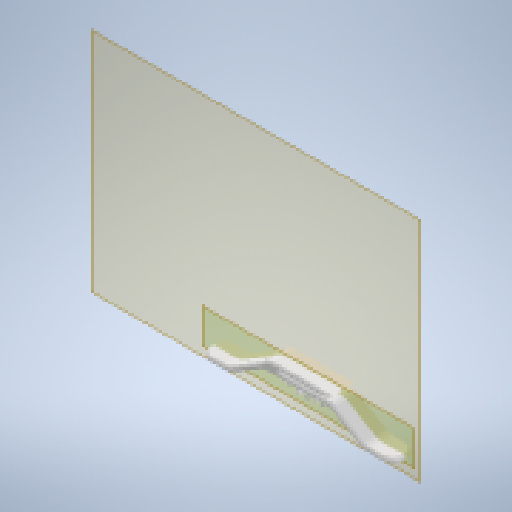
# Autodesk Inventor part: cable-hanger
Saved by Autodesk Inventor 2023 (Build 270158030, 158C)
## iProperties
Created: 2024-09-24
Part Number: cable-hanger
Material: Generic
Document SubType Name: Modeling
Designer: Imogen Heard
Density: 1 g/cm^3
Appearance: Default
Author: Imogen Heard
Autodesk Inventor part; units mm, degrees
ref_plane "YZ Plane" through (0, 0, 0) normal (1, 0, 0) x (0, 1, 0)
ref_plane "XZ Plane" through (0, 0, 0) normal (0, 1, 0) x (-1, 0, 0)
ref_plane "XY Plane" through (0, 0, 0) normal (0, 0, 1) x (1, 0, 0)
sketch "Sketch1" plane through (0, 0, 0) normal (0, 0, 1) x (1, 0, 0)
  line L0 (-0.831, -6.5) -> (-20.831, -6.5)
  line L1 (-20.831, -6.5) -> (-20.831, -3.5)
  line L2 (-20.831, -3.5) -> (0, -3.5)
  line L3 (0, -3.5) -> (20, -15.5)
  line L4 (20, -15.5) -> (36.169, -15.5)
  line L5 (36.169, -15.5) -> (36.169, -18.5)
  line L6 (36.169, -18.5) -> (19.169, -18.5)
  line L7 (19.169, -18.5) -> (-0.831, -6.5)
  line L8 (-40.831, -6.5) -> (-20.831, -6.5)
  line L9 (-20.831, -3.5) -> (-41.6619, -3.5)
  line L10 (-41.6619, -3.5) -> (-61.6619, -15.5)
  line L11 (-61.6619, -15.5) -> (-77.831, -15.5)
  line L12 (-77.831, -15.5) -> (-77.831, -18.5)
  line L13 (-77.831, -18.5) -> (-60.831, -18.5)
  line L14 (-60.831, -18.5) -> (-40.831, -6.5)
  line L15 (-41.6619, -3.5) -> (-31.6619, -3.5)
  line L16 (-31.6619, -3.5) -> (-31.6619, -2)
  line L17 (-31.6619, -2) -> (-41.6619, -2)
  line L18 (-41.6619, -2) -> (-41.6619, -3.5)
  line L19 (-41.6619, -2) -> (0, -2)
  line L20 (0, -2) -> (0, 0)
  line L21 (0, 0) -> (-41.6619, 0)
  line L22 (-41.6619, 0) -> (-41.6619, -2)
  point P0 (65.831, 133)
  point P1 (105.831, 133)
  point P2 (106.6619, 130)
  point P3 (96.6619, 130)
  point P4 (96.6619, 128.5)
  dimension "d0" = 3
  dimension "d1" = 3
  dimension "d2" = 3
  dimension "d3" = 17
  dimension "d4" = -20
  dimension "d5" = -12
  dimension "d6" = 20
  dimension "d7" = 114
  dimension "d8" = 20
  dimension "d9" = -20
  dimension "d10" = 17
  dimension "d11" = 2
  dimension "d12" = 1.5
  dimension "d13" = 10
  constraints: 46 end point, 7 symmetric about line, 6 parallel, 5 perpendicular, 2 coincident, 1 horizontal alignment, 1 vertical alignment
  measures "d0" distance between parallel lines of L2 L0
  measures "d1" distance between parallel lines of L3 L7
  measures "d2" distance between parallel lines of L4 L6
  measures "d3" distance from line of L5 L6.end
  measures "d4" horizontal distance of L0.start L6.end
  measures "d5" vertical distance of L0.start L6.end
  measures "d6" distance of L0.start L0.end
  measures "d7" distance between parallel lines of L12 L5
  measures "d8" distance from line of L8.start L1
  measures "d9" horizontal distance of L13.end L14.end
  measures "d10" distance of L12.end L13.end
  measures "d11" distance between parallel lines of L21 L19
  measures "d12" distance between parallel lines of L19 L9
  measures "d13" distance between parallel lines of L16 L22
extrude "Extrusion1" add sketch "Sketch1" along normal blind 15
fillet "Fillet1" radius 7.5 4 edges at (-77.831, -17, 0) (-77.831, -17, 15) (36.169, -17, 15) (36.169, -17, 0)
fillet "Fillet2" radius 10 9 edges at (-41.6619, 0, 7.5) (-61.6619, -15.5, 7.5) (-60.831, -18.5, 7.5) (-40.831, -6.5, 7.5) (-0.831, -6.5, 7.5) (19.169, -18.5, 7.5) (20, -15.5, 7.5) (0, -3.5, 7.5) (0, -2, 7.5)
chamfer "Chamfer1" distance 1 angle 45 50 edges at (-20.831, -6.5, 0) (-0.9315, -6.8629, 0) (9.169, -12.5, 0) (19.2696, -18.1371, 0) (25.304, -18.5, 0) (33.9724, -18.5, 2.1967) (36.169, -18.5, 7.5) (33.9724, -18.5, 12.8033) (25.304, -18.5, 15) (19.2696, -18.1371, 15) (9.169, -12.5, 15) (-0.9315, -6.8629, 15) (-20.831, -6.5, 15) (-40.7304, -6.8629, 15) (-50.831, -12.5, 15) (-60.9315, -18.1371, 15) (-66.9659, -18.5, 15) (-75.6343, -18.5, 2.1967) (-77.831, -18.5, 7.5) (-75.6343, -18.5, 12.8033) (-66.9659, -18.5, 0) (-60.9315, -18.1371, 0) (-50.831, -12.5, 0) (-40.7304, -6.8629, 0) (-50.4743, -8.7875, 15) (-61.7624, -15.1371, 15) (-67.3814, -15.5, 15) (-75.6343, -15.5, 2.1967) (-77.831, -15.5, 7.5) (-75.6343, -15.5, 12.8033) (-67.3814, -15.5, 0) (-61.7624, -15.1371, 0) (-50.4743, -8.7875, 0) (-38.2459, -0.917, 15) (-17.0313, 0, 15) (-38.2459, -0.917, 0) (-17.0313, 0, 0) (25.7195, -15.5, 15) (20.1005, -15.1371, 15) (10, -9.5, 15) (-0.1005, -3.8629, 15) (-17.2159, -3.5, 15) (33.9724, -15.5, 2.1967) (36.169, -15.5, 7.5) (33.9724, -15.5, 12.8033) (25.7195, -15.5, 0) (20.1005, -15.1371, 0) (10, -9.5, 0) (-0.1005, -3.8629, 0) (-17.2159, -3.5, 0)
ref_plane "Work Plane1" through (0, 0, 7.5) normal (0, 0, 1) x (1, 0, 0)
sketch "Sketch2" plane through (0, 0, 7.5) normal (0, 0, 1) x (1, 0, 0)
  circle A0 centre (-135.4999, 85.8508) radius 2.5
  circle A1 centre (-134.65, 75.8508) radius 1.65
  line L0 (-133, 103.0611) -> (-133, 68.6008)
  circle A2 centre (-135, 95.8508) radius 2
  circle A3 centre (-134.65, 75.8508) radius 2.85
  circle A4 centre (-135.4999, 85.8508) radius 3.7
  circle A5 centre (-135, 95.8508) radius 3.2
  line L1 (-137.9999, 75.0258) -> (-135.6676, 75.0258)
  line L2 (-135.6676, 75.0258) -> (-135.6676, 76.6758)
  line L3 (-135.6676, 76.6758) -> (-137.9999, 76.6758)
  line L4 (-137.9999, 76.6758) -> (-137.9999, 75.0258)
  line L5 (-139.843, 84.6008) -> (-137.5, 84.6008)
  line L6 (-137.5, 84.6008) -> (-137.5, 87.1008)
  line L7 (-137.5, 87.1008) -> (-139.843, 87.1008)
  line L8 (-139.843, 87.1008) -> (-139.843, 84.6008)
  line L9 (-138.6715, 94.8508) -> (-136.0812, 94.8508)
  line L10 (-136.0812, 94.8508) -> (-136.0812, 96.8508)
  line L11 (-136.0812, 96.8508) -> (-138.6715, 96.8508)
  line L12 (-138.6715, 96.8508) -> (-138.6715, 94.8508)
  circle A6 centre (-135.4999, 85.8508) radius 2.5
  circle A7 centre (-134.65, 75.8508) radius 1.65
  line L13 (-133, 103.0611) -> (-133, 68.6008)
  circle A8 centre (-135, 95.8508) radius 2
  circle A9 centre (-134.65, 75.8508) radius 2.85
  circle A10 centre (-135.4999, 85.8508) radius 3.7
  circle A11 centre (-135, 95.8508) radius 3.2
  line L14 (-137.9999, 75.0258) -> (-135.6676, 75.0258)
  line L15 (-135.6676, 75.0258) -> (-135.6676, 76.6758)
  line L16 (-135.6676, 76.6758) -> (-137.9999, 76.6758)
  line L17 (-137.9999, 76.6758) -> (-137.9999, 75.0258)
  line L18 (-139.843, 84.6008) -> (-137.5, 84.6008)
  line L19 (-137.5, 84.6008) -> (-137.5, 87.1008)
  line L20 (-137.5, 87.1008) -> (-139.843, 87.1008)
  line L21 (-139.843, 87.1008) -> (-139.843, 84.6008)
  line L22 (-138.6715, 94.8508) -> (-136.0812, 94.8508)
  line L23 (-136.0812, 94.8508) -> (-136.0812, 96.8508)
  line L24 (-136.0812, 96.8508) -> (-138.6715, 96.8508)
  line L25 (-138.6715, 96.8508) -> (-138.6715, 94.8508)
  circle A12 centre (-11.331, -9) radius 2.5
  circle A13 centre (-20.831, -9.5) radius 3
  circle A14 centre (-30.331, -8.5) radius 2
  line L26 (28.669, -16.5) -> (28.669, -16.5) projected
  line L27 (28.669, -16.5) -> (28.669, -17.5) projected
  line L28 (28.669, -17.5) -> (28.669, -17.5) projected
  line L29 (28.669, -17.5) -> (28.669, -16.5) projected
  line L30 (22.7698, -16.5) -> (28.669, -16.5) projected
  arc A15 (17.1104, -14.9324) -> (22.7698, -16.5) centre (22.7698, -5.5) ccw projected
  line L31 (1.8606, -5.7826) -> (17.1104, -14.9324) projected
  arc A16 (1.8606, -5.7826) -> (-2.7698, -4.5) centre (-2.7698, -13.5) ccw projected
  line L32 (-31.6619, -4.5) -> (-2.7698, -4.5) projected
  line L33 (-31.6619, -4.5) -> (-31.6619, -2) projected
  line L34 (-31.6619, -2) -> (-6, -2) projected
  arc A17 (-6, -2) -> (-1.6411, -1) centre (-6, 8) ccw projected
  line L35 (-34.0626, -1) -> (-1.6411, -1) projected
  arc A18 (-34.0626, -1) -> (-41.004, -4.2715) centre (-34.0626, -10) ccw projected
  line L36 (-58.7723, -14.9324) -> (-41.004, -4.2715) projected
  arc A19 (-64.4317, -16.5) -> (-58.7723, -14.9324) centre (-64.4317, -5.5) ccw projected
  line L37 (-70.331, -16.5) -> (-64.4317, -16.5) projected
  line L38 (-70.331, -17.5) -> (-70.331, -16.5) projected
  line L39 (-63.6008, -17.5) -> (-70.331, -17.5) projected
  arc A20 (-63.6008, -17.5) -> (-58.9703, -16.2174) centre (-63.6008, -8.5) ccw projected
  line L40 (-43.7206, -7.0676) -> (-58.9703, -16.2174) projected
  arc A21 (-38.0611, -5.5) -> (-43.7206, -7.0676) centre (-38.0611, -16.5) ccw projected
  line L41 (-3.6008, -5.5) -> (-38.0611, -5.5) projected
  arc A22 (2.0587, -7.0676) -> (-3.6008, -5.5) centre (-3.6008, -16.5) ccw projected
  line L42 (17.3084, -16.2174) -> (2.0587, -7.0676) projected
  arc A23 (17.3084, -16.2174) -> (21.9389, -17.5) centre (21.9389, -8.5) ccw projected
  line L43 (28.669, -17.5) -> (21.9389, -17.5) projected
  line L44 (28.669, -16.5) -> (28.669, -17.5) projected
  line L45 (-38.0611, -6.5) -> (-3.6008, -6.5) projected
  line L46 (-38.0611, -6.5) -> (-3.6008, -6.5) projected
  line L47 (-3.6008, -6.5) -> (-38.0611, -6.5) projected
  circle A24 centre (-11.331, -9) radius 3.7
  circle A25 centre (-20.831, -9.5) radius 4.2
  circle A26 centre (-30.331, -8.5) radius 3.2
  line L48 (-10.081, -12.8117) -> (-12.581, -12.8117)
  line L49 (-12.581, -12.8117) -> (-12.581, -9.85)
  line L50 (-12.581, -9.85) -> (-10.081, -9.85)
  line L51 (-10.081, -9.85) -> (-10.081, -12.8117)
  line L52 (-19.331, -14.2793) -> (-22.331, -14.2793)
  line L53 (-22.331, -14.2793) -> (-22.331, -10.8575)
  line L54 (-22.331, -10.8575) -> (-19.331, -10.8575)
  line L55 (-19.331, -10.8575) -> (-19.331, -14.2793)
  line L56 (-29.331, -12.7) -> (-31.331, -12.7)
  line L57 (-31.331, -12.7) -> (-31.331, -9.3912)
  line L58 (-31.331, -9.3912) -> (-29.331, -9.3912)
  line L59 (-29.331, -9.3912) -> (-29.331, -12.7)
  point P0 (0, 0)
  point P1 (-130, 65)
  point P2 (-133, 85.831)
  point P3 (-130, 65)
  point P4 (-133, 85.831)
  point P5 (-29.331, -10.2321)
  point P6 (-29.331, -11.5397)
  point P7 (-27.833, -6.5)
  point P8 (-30.331, -6.5)
  point P9 (-31.331, -11.5397)
  point P10 (-31.331, -10.2321)
  point P11 (-32.829, -6.5)
  point P12 (-19.331, -12.0981)
  point P13 (-19.331, -13.423)
  point P14 (-17.8916, -6.5)
  point P15 (-20.831, -6.5)
  point P16 (-22.331, -13.423)
  point P17 (-22.331, -12.0981)
  point P18 (-23.7703, -6.5)
  point P19 (-10.081, -11.1651)
  point P20 (-10.081, -12.4825)
  point P21 (-10.131, -5.5)
  point P22 (-31.4445, -5.5)
  point P23 (-29.2174, -5.5)
  point P24 (-22.1116, -5.5)
  point P25 (-19.5503, -5.5)
  point P26 (-12.531, -5.5)
  point P27 (-12.581, -12.4825)
  point P28 (-12.581, -11.1651)
  dimension "d27" = 5
  dimension "d43" = 5
  dimension "d21" = 10
  dimension "d22" = 10
  dimension "d23" = 7.2103
  dimension "d24" = 7.25
  dimension "d25" = 3.3
  dimension "d26" = 4
  dimension "d28" = 1.2
  dimension "d29" = 1.2
  dimension "d30" = 1.2
  dimension "d31" = 2.5
  dimension "d32" = 1.25
  dimension "d33" = 1.65
  dimension "d34" = 0.825
  dimension "d35" = 2
  dimension "d36" = 1
  dimension "d37" = 10
  dimension "d38" = 10
  dimension "d39" = 7.2103
  dimension "d40" = 7.25
  dimension "d41" = 3.3
  dimension "d42" = 4
  dimension "d44" = 1.2
  dimension "d45" = 1.2
  dimension "d46" = 1.2
  dimension "d47" = 2.5
  dimension "d48" = 1.25
  dimension "d49" = 1.65
  dimension "d50" = 0.825
  dimension "d51" = 2
  dimension "d52" = 1
  dimension "d53" = 5
  dimension "d54" = 6
  dimension "d55" = 4
  dimension "d56" = 40
  dimension "d57" = 40
  dimension "d58" = 9.5
  dimension "d59" = 9.5
  dimension "d60" = 1.2
  dimension "d61" = 1.2
  dimension "d62" = 1.2
  dimension "d63" = 2.5
  dimension "d64" = 1.25
  dimension "d65" = 3
  dimension "d66" = 1.5
  dimension "d67" = 2
  dimension "d68" = 1
  constraints: 76 end point, 18 parallel, 16 centre point, 9 horizontal, 9 perpendicular, 7 tangent, 2 midpoint, 6 other
  measures "d21" vertical distance of A4.centre A1.centre
  measures "d22" vertical distance of A2.centre A4.centre
  measures "d23" vertical distance of L0.start A2.centre
  measures "d24" vertical distance of A1.centre L0.end
  measures "d25" diameter of A1
  measures "d26" diameter of A2
  measures "d29" radial gap between concentric circles of A5 A2
  measures "d30" radial gap between concentric circles of A3 A1
  measures "d31" distance between parallel lines of L7 L5
  measures "d32" distance from line of A4.centre L5
  measures "d33" distance between parallel lines of L3 L1
  measures "d34" distance from line of L1 A1.centre
  measures "d35" distance between parallel lines of L11 L9
  measures "d36" distance from line of L9 A2.centre
  measures "d37" vertical distance of A10.centre A7.centre
  measures "d38" vertical distance of A8.centre A10.centre
  measures "d39" vertical distance of L13.start A8.centre
  measures "d40" vertical distance of A7.centre L13.end
  measures "d41" diameter of A7
  measures "d42" diameter of A8
  measures "d45" radial gap between concentric circles of A11 A8
  measures "d46" radial gap between concentric circles of A9 A7
  measures "d47" distance between parallel lines of L20 L18
  measures "d48" distance from line of A10.centre L18
  measures "d49" distance between parallel lines of L16 L14
  measures "d50" distance from line of L14 A7.centre
  measures "d51" distance between parallel lines of L24 L22
  measures "d52" distance from line of L22 A8.centre
  measures "d53" diameter of A12
  measures "d54" diameter of A13
  measures "d55" diameter of A14
  measures "d56" distance from line of A14.centre L38
  measures "d57" distance from line of L27 A12.centre
  measures "d58" horizontal distance of A13.centre A12.centre
  measures "d59" horizontal distance of A14.centre A13.centre
  measures "d60" radial gap between concentric circles of A24 A12
  measures "d61" radial gap between concentric circles of A25 A13
  measures "d62" radial gap between concentric circles of A14 A26
  measures "d63" distance between parallel lines of L49 L51
  measures "d64" distance from line of L51 A12.centre
  measures "d65" distance between parallel lines of L53 L55
  measures "d66" distance from line of L55 A13.centre
  measures "d67" distance between parallel lines of L57 L59
  measures "d68" distance from line of L59 A14.centre
extrude "Extrusion2" add sketch "Sketch2" along normal mid plane 8 contours A12 L45 A24 L51 | A12 L49 A24 L45 | L45 A24 L41 | A25 L55 A13 L45 | A24 L41 | L41 A25 A26 A21 L40 A20 L39 L38 L37 A19 L36 A18 L35 A17 L34 L33 L32 A16 L31 A15 L30 L27 L43 A23 L42 A22 A24 | A13 L53 A25 L45 | A26 L59 A14 L45 | A14 L57 A26 L45
fillet "Fillet3" radius 1 6 edges at (-8.6033, -6.5, 7.5) (-14.0586, -6.5, 7.5) (-17.8916, -6.5, 7.5) (-23.7703, -6.5, 7.5) (-27.833, -6.5, 7.5) (-32.829, -6.5, 7.5)
fillet "Fillet4" radius 1 6 edges at (-10.081, -12.4825, 7.5) (-12.581, -12.4825, 7.5) (-19.331, -13.423, 7.5) (-22.331, -13.423, 7.5) (-29.331, -11.5397, 7.5) (-31.331, -11.5397, 7.5)
chamfer "Chamfer2" distance 1 angle 45 12 edges at (-23.231, -6.5, 3.5) (-18.431, -6.5, 3.5) (-13.5581, -6.5, 3.5) (-9.1038, -6.5, 3.5) (-28.2913, -6.5, 3.5) (-32.3706, -6.5, 3.5) (-32.3706, -6.5, 11.5) (-28.2913, -6.5, 11.5) (-23.231, -6.5, 11.5) (-18.431, -6.5, 11.5) (-13.5581, -6.5, 11.5) (-9.1038, -6.5, 11.5)
ref_plane "Work Plane2" through (0, 0, 7.5) normal (0, 0, -1) x (-1, 0, 0)
sketch "Sketch3" plane through (0, 0, 7.5) normal (0, 0, -1) x (-1, 0, 0)
  arc A0 (1.6411, -1) -> (6, -2) centre (6, 8) ccw projected
  circle A1 centre (3.75, -1.7436) radius 0.75
  line L0 (27.1619, -2.2) -> (4.5, -2.2) projected
  line L1 (4.5, -2.2) -> (4.5, -3.5) projected
  point P0 (0, 0)
  point P1 (4.4866, -1.8848)
  point P2 (3.0261, -1.5476)
  dimension "d76" = 1.5
  dimension "d77" = 0.75
  constraints: 1 centre point, 1 point on circle
  measures "d76" diameter of A1
  measures "d77" distance from line of L1 A1.centre
extrude "Extrusion3" add sketch "Sketch3" along normal mid plane 8 contours A0 A1 picked at (3.7247, -1.9902)
chamfer "Chamfer3" distance 0.749 angle 45 2 edges at (-3.75, -1.7436, 3.5) (-3.75, -1.7436, 11.5)
chamfer "Chamfer4" distance 0.5 angle 45 36 edges at (-32.1702, -10.6978, 3.5) (-33.4861, -9.034, 3.5) (-33.4174, -7.6199, 3.5) (-28.4917, -10.6978, 3.5) (-27.1758, -9.034, 3.5) (-27.2445, -7.6199, 3.5) (-23.0936, -12.6256, 3.5) (-24.9722, -10.1999, 3.5) (-24.6504, -7.6961, 3.5) (-18.5683, -12.6256, 3.5) (-16.6897, -10.1999, 3.5) (-17.0115, -7.6961, 3.5) (-7.6852, -9.6314, 3.5) (-9.287, -11.6691, 3.5) (-7.8636, -7.6617, 3.5) (-13.3749, -11.6691, 3.5) (-14.9767, -9.6314, 3.5) (-14.7983, -7.6617, 3.5) (-9.287, -11.6691, 11.5) (-7.6852, -9.6314, 11.5) (-7.8636, -7.6617, 11.5) (-13.3749, -11.6691, 11.5) (-14.9767, -9.6314, 11.5) (-14.7983, -7.6617, 11.5) (-16.6897, -10.1999, 11.5) (-17.0115, -7.6961, 11.5) (-18.5683, -12.6256, 11.5) (-23.0936, -12.6256, 11.5) (-24.9722, -10.1999, 11.5) (-24.6504, -7.6961, 11.5) (-28.4917, -10.6978, 11.5) (-27.1758, -9.034, 11.5) (-27.2445, -7.6199, 11.5) (-32.1702, -10.6978, 11.5) (-33.4861, -9.034, 11.5) (-33.4174, -7.6199, 11.5)
equation "\"d1\" = d0"
equation "\"d2\" = d1"
equation "\"d29\" = d28"
equation "\"d30\" = d28"
equation "\"d31\" = 0.5 * d27"
equation "\"d32\" = 0.5 * d31"
equation "\"d33\" = 0.5 * d25"
equation "\"d34\" = 0.5 * d33"
equation "\"d35\" = 0.5 * d26"
equation "\"d36\" = 0.5 * d35"
equation "\"d45\" = d44"
equation "\"d46\" = d44"
equation "\"d47\" = 0.5 * d43"
equation "\"d48\" = 0.5 * d47"
equation "\"d49\" = 0.5 * d41"
equation "\"d50\" = 0.5 * d49"
equation "\"d51\" = 0.5 * d42"
equation "\"d52\" = 0.5 * d51"
equation "\"d57\" = d56"
